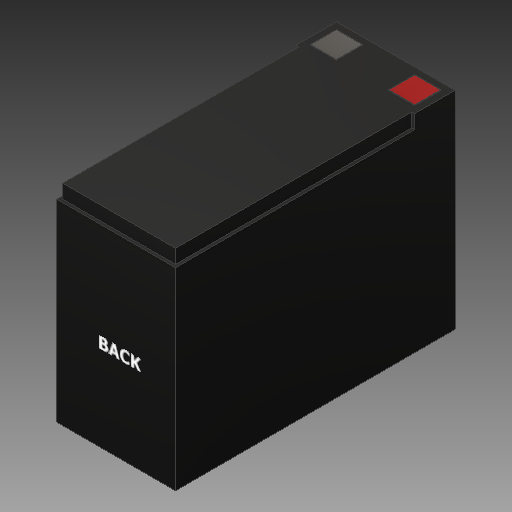
# Autodesk Inventor part: BotBattery
Saved by Autodesk Inventor 2019 (Build 230136000, 136)
## iProperties
Created: 2016-08-31
Part Number: BotBattery
Material: Generic
Document SubType Name: Modeling
Designer: budak7273
Density: 1 g/cm^3
Appearance: Default
Mass: 1049.18 g
Surface Area: 662.409 cm^2
Volume: 1049.18 cm^3
Author: budak7273
Autodesk Inventor part; units mm, degrees
ref_plane "YZ Plane" through (0, 0, 0) normal (1, 0, 0) x (0, 1, 0)
ref_plane "XZ Plane" through (0, 0, 0) normal (0, 1, 0) x (-1, 0, 0)
ref_plane "XY Plane" through (0, 0, 0) normal (0, 0, 1) x (1, 0, 0)
sketch "Sketch1" plane through (0, 0, 0) normal (0, 1, 0) x (-1, 0, 0)
  line L0 (31.75, 74.8157) -> (-31.75, 74.8157)
  line L1 (-31.75, 74.8157) -> (-31.75, -74.8157)
  line L2 (-31.75, -74.8157) -> (31.75, -74.8157)
  line L3 (31.75, -74.8157) -> (31.75, 74.8157)
  line L4 (0, 0) -> (31.75, 0) construction
  line L5 (0, 0) -> (0, 74.8157) construction
  line L6 (0, 0) -> (-31.75, 0) construction
  line L7 (0, 0) -> (0, -74.8157) construction
  dimension "d0" = 63.5
  dimension "d1" = 149.6314
  constraints: 16 end point, 4 midpoint, 3 perpendicular, 2 collinear, 2 parallel, 2 point on line, 1 horizontal
  measures "d0" distance of L2.end L1.end
  measures "d1" distance of L1.end L0.end
extrude "Extrusion1" add sketch "Sketch1" along normal blind 110.8075
sketch "Sketch2" plane through (0, 110.8075, 0) normal (0, 1, 0) x (1, 0, 0)
  line L0 (-31.75, -74.8157) -> (31.75, -74.8157) projected
  line L1 (31.75, -74.8157) -> (31.75, 74.8157) projected
  line L2 (31.75, 74.8157) -> (-31.75, 74.8157) projected
  line L3 (-31.75, 74.8157) -> (-31.75, -74.8157) projected
  line L4 (-30.1498, -73.2155) -> (30.1498, -73.2155)
  line L5 (30.1498, -73.2155) -> (30.1498, 73.2155)
  line L6 (30.1498, 73.2155) -> (-30.1498, 73.2155)
  line L7 (-30.1498, 73.2155) -> (-30.1498, -73.2155)
  point P0 (0, 0)
  dimension "d4" = 1.6002
  constraints: 8 end point, 3 other
  measures "d4" distance between parallel lines of L3 L7
extrude "Extrusion2" cut sketch "Sketch2" against normal blind 7.4422
sketch "Sketch3" plane through (0, 103.3653, 0) normal (0, 1, 0) x (1, 0, 0)
  line L0 (-30.1498, 73.2155) -> (-30.1498, 53.2257)
  line L1 (30.1498, 73.2155) -> (-30.1498, 73.2155)
  line L2 (31.75, 74.8157) -> (31.75, 53.2257)
  line L3 (-31.75, 74.8157) -> (31.75, 74.8157)
  line L4 (30.1498, 73.2155) -> (-30.1498, 73.2155) projected
  line L5 (-31.75, 53.2257) -> (-30.1498, 53.2257)
  line L6 (31.75, 53.2257) -> (30.1498, 53.2257)
  line L7 (30.1498, 53.2257) -> (30.1498, 73.2155)
  line L8 (-31.75, 53.2257) -> (-31.75, 74.8157)
  point P0 (0, 0)
  dimension "d7" = 21.59
  constraints: 16 end point, 5 perpendicular, 2 equal length, 1 horizontal
  measures "d7" distance between parallel lines of L3 L5
sketch "Sketch4" plane through (0, 103.3653, 0) normal (0, 1, 0) x (1, 0, 0)
  line L0 (-31.75, 74.8157) -> (31.75, 74.8157) projected
  line L1 (30.1498, 73.2155) -> (-30.1498, 73.2155) projected
  line L2 (-31.75, 74.8157) -> (-31.75, 53.2257)
  line L3 (-31.75, 53.2257) -> (-30.1498, 53.2257)
  line L4 (-30.1498, 73.2155) -> (-30.1498, 53.2257)
  line L5 (0, 73.2155) -> (0, 74.8157) construction
  line L6 (31.75, 74.8157) -> (31.75, 53.2257)
  line L7 (31.75, 53.2257) -> (30.1498, 53.2257)
  line L8 (30.1498, 73.2155) -> (30.1498, 53.2257)
  point P0 (0, 0)
  dimension "d8" = 21.59
  constraints: 14 end point, 2 midpoint, 2 perpendicular, 2 symmetric about line, 1 horizontal
  measures "d8" distance of L0.start L2.end
extrude "Extrusion3" add sketch "Sketch4" along normal up to surface (7.4422 mm away)
sketch "Sketch5" plane through (-31.75, 0, 74.8157) normal (0, 0, 1) x (1, 0, 0)
  line L0 (22.0103, 51.8449) -> (31.9769, 51.8449) construction
  line L1 (31.9769, 51.8449) -> (31.9769, 48.6882) construction
  line L2 (31.9769, 48.6882) -> (22.0103, 48.6882) construction
  line L3 (22.0103, 48.6882) -> (22.0103, 51.8449) construction
  constraints: 2 other
sketch "Sketch6" plane through (31.75, 0, -74.8157) normal (0, 0, -1) x (-1, 0, 0)
  line L0 (18.5743, 56.7919) -> (44.5786, 56.7919) construction
  line L1 (44.5786, 56.7919) -> (44.5786, 50.439) construction
  line L2 (44.5786, 50.439) -> (18.5743, 50.439) construction
  line L3 (18.5743, 50.439) -> (18.5743, 56.7919) construction
  constraints: 2 other
sketch "Sketch7" plane through (0, 110.8075, 0) normal (0, 1, 0) x (1, 0, 0)
  line L0 (27.94, 71.0057) -> (13.97, 71.0057)
  line L1 (13.97, 71.0057) -> (13.97, 57.0357)
  line L2 (13.97, 57.0357) -> (27.94, 57.0357)
  line L3 (27.94, 57.0357) -> (27.94, 71.0057)
  line L4 (31.75, 74.8157) -> (31.75, 53.2257) construction
  line L5 (-31.75, 74.8157) -> (31.75, 74.8157) construction
  line L6 (0, 74.8157) -> (0, -73.2155) construction
  line L7 (-30.1498, -73.2155) -> (30.1498, -73.2155) construction
  line L8 (-27.94, 71.0057) -> (-13.97, 71.0057)
  line L9 (-13.97, 71.0057) -> (-13.97, 57.0357)
  line L10 (-13.97, 57.0357) -> (-27.94, 57.0357)
  line L11 (-27.94, 57.0357) -> (-27.94, 71.0057)
  point P0 (0, 0)
  dimension "d11" = 13.97
  dimension "d12" = 3.81
  dimension "d13" = 3.81
  constraints: 18 end point, 4 symmetric about line, 2 midpoint, 2 parallel, 2 perpendicular, 1 horizontal
  measures "d11" distance of L2.end L0.start
  measures "d12" distance between parallel lines of L4 L3
  measures "d13" distance between parallel lines of L5 L0
extrude "Extrusion4" add sketch "Sketch7" along normal blind 0.254
equation "\"d13\" = d12"
body "Solid1"
